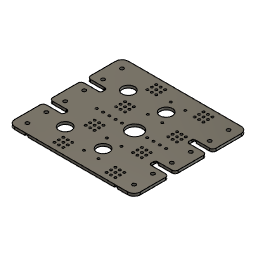
JumperTrunk_TopPlate_4mm v2 (Autodesk Fusion 360 design; units mm, degrees)
Autodesk Fusion 360 part; units mm, degrees
(part 1 of 2)
sketch "Sketch1" plane through (0, 0, 0) normal (0, 1, 0) x (1, 0, 0)
  arc A0 (10, 180) -> (0, 170) centre (10, 170) ccw
  circle A1 centre (15, 105) radius 2.75
  line L0 (171, 125) -> (194, 125)
  line L1 (199, 150) -> (199, 170)
  circle A2 centre (184, 165) radius 2.75
  arc A3 (189, 0) -> (199, 10) centre (189, 10) ccw
  line L2 (0, 150) -> (0, 170)
  circle A4 centre (184, 135) radius 2.75
  line L3 (199, 30) -> (199, 10)
  line L4 (168, 58) -> (168, 62)
  circle A5 centre (184, 105) radius 2.75
  line L5 (194, 55) -> (171, 55)
  line L6 (5, 115) -> (28, 115)
  circle A6 centre (15, 15) radius 2.75
  line L7 (0, 142) -> (0, 142.1084)
  circle A7 centre (184, 45) radius 2.75
  line L8 (0, 30) -> (0, 10)
  arc A8 (0, 10) -> (10, 0) centre (10, 10) ccw
  line L9 (31, 118) -> (31, 122)
  line L10 (5, 55) -> (28, 55)
  circle A9 centre (15, 135) radius 2.75
  line L11 (0, 82) -> (0, 82.1084)
  circle A10 centre (15, 165) radius 2.75
  line L12 (28, 65) -> (5, 65)
  line L13 (31, 58) -> (31, 62)
  circle A11 centre (15, 45) radius 2.75
  line L14 (0, 52) -> (0, 52.1084)
  line L15 (171, 65) -> (194, 65)
  line L16 (28, 125) -> (5, 125)
  circle A12 centre (184, 15) radius 2.75
  line L17 (0, 112) -> (0, 112.1084)
  line L18 (168, 118) -> (168, 122)
  line L19 (194, 115) -> (171, 115)
  line L20 (10, 0) -> (189, 0)
  line L21 (10, 180) -> (189, 180)
  arc A13 (199, 170) -> (189, 180) centre (189, 170) ccw
  circle A14 centre (70, 17) radius 1.75
  circle A15 centre (71.3, 65.26) radius 1.75
  circle A16 centre (146.23, 65.26) radius 1.75
  circle A17 centre (152.55, 17) radius 1.75
  circle A18 centre (70, 17) radius 1.75
  circle A19 centre (146.23, 65.26) radius 1.75
  circle A20 centre (71.3, 65.26) radius 1.75
  circle A21 centre (152.55, 17) radius 1.75
  circle A22 centre (71.3, 65.26) radius 1.75
  circle A23 centre (152.55, 17) radius 1.75
  circle A24 centre (146.23, 65.26) radius 1.75
  circle A25 centre (152.55, 17) radius 1.75
  circle A26 centre (70, 17) radius 1.75
  circle A27 centre (71.3, 65.26) radius 1.75
  circle A28 centre (146.23, 65.26) radius 1.75
  circle A29 centre (70, 17) radius 1.75
  circle A30 centre (64.3, 58.26) radius 1.75
  circle A31 centre (71.3, 58.26) radius 1.75
  circle A32 centre (78.3, 58.26) radius 1.75
  circle A33 centre (64.3, 65.26) radius 1.75
  circle A34 centre (78.3, 65.26) radius 1.75
  circle A35 centre (64.3, 72.26) radius 1.75
  circle A36 centre (71.3, 72.26) radius 1.75
  circle A37 centre (78.3, 72.26) radius 1.75
  circle A38 centre (63, 10) radius 1.75
  circle A39 centre (70, 10) radius 1.75
  circle A40 centre (77, 10) radius 1.75
  circle A41 centre (63, 17) radius 1.75
  circle A42 centre (77, 17) radius 1.75
  circle A43 centre (63, 24) radius 1.75
  circle A44 centre (70, 24) radius 1.75
  circle A45 centre (77, 24) radius 1.75
  circle A46 centre (139.23, 58.26) radius 1.75
  circle A47 centre (146.23, 58.26) radius 1.75
  circle A48 centre (153.23, 58.26) radius 1.75
  circle A49 centre (139.23, 65.26) radius 1.75
  circle A50 centre (153.23, 65.26) radius 1.75
  circle A51 centre (139.23, 72.26) radius 1.75
  circle A52 centre (146.23, 72.26) radius 1.75
  circle A53 centre (153.23, 72.26) radius 1.75
  circle A54 centre (145.55, 10) radius 1.75
  circle A55 centre (152.55, 10) radius 1.75
  circle A56 centre (159.55, 10) radius 1.75
  circle A57 centre (145.55, 17) radius 1.75
  circle A58 centre (159.55, 17) radius 1.75
  circle A59 centre (145.55, 24) radius 1.75
  circle A60 centre (152.55, 24) radius 1.75
  circle A61 centre (159.55, 24) radius 1.75
  circle A62 centre (159.55, 24) radius 1.75
  circle A63 centre (153.23, 65.26) radius 1.75
  circle A64 centre (71.3, 65.26) radius 1.75
  circle A65 centre (71.3, 65.26) radius 1.75
  circle A66 centre (70, 17) radius 1.75
  circle A67 centre (71.3, 72.26) radius 1.75
  circle A68 centre (146.23, 65.26) radius 1.75
  circle A69 centre (152.55, 17) radius 1.75
  circle A70 centre (63, 17) radius 1.75
  circle A71 centre (78.3, 65.26) radius 1.75
  circle A72 centre (146.23, 65.26) radius 1.75
  circle A73 centre (70, 17) radius 1.75
  circle A74 centre (159.55, 17) radius 1.75
  circle A75 centre (146.23, 72.26) radius 1.75
  circle A76 centre (153.23, 72.26) radius 1.75
  circle A77 centre (71.3, 65.26) radius 1.75
  circle A78 centre (139.23, 65.26) radius 1.75
  circle A79 centre (63, 24) radius 1.75
  circle A80 centre (77, 24) radius 1.75
  circle A81 centre (139.23, 72.26) radius 1.75
  circle A82 centre (64.3, 65.26) radius 1.75
  circle A83 centre (71.3, 65.26) radius 1.75
  circle A84 centre (71.3, 58.26) radius 1.75
  circle A85 centre (145.55, 24) radius 1.75
  circle A86 centre (152.55, 17) radius 1.75
  circle A87 centre (70, 17) radius 1.75
  circle A88 centre (70, 17) radius 1.75
  circle A89 centre (77, 17) radius 1.75
  circle A90 centre (64.3, 72.26) radius 1.75
  circle A91 centre (77, 10) radius 1.75
  circle A92 centre (152.55, 17) radius 1.75
  circle A93 centre (64.3, 58.26) radius 1.75
  circle A94 centre (145.55, 17) radius 1.75
  circle A95 centre (70, 24) radius 1.75
  circle A96 centre (63, 10) radius 1.75
  circle A97 centre (70, 10) radius 1.75
  circle A98 centre (159.55, 10) radius 1.75
  circle A99 centre (145.55, 10) radius 1.75
  circle A100 centre (152.55, 24) radius 1.75
  circle A101 centre (152.55, 10) radius 1.75
  circle A102 centre (152.55, 17) radius 1.75
  circle A103 centre (139.23, 58.26) radius 1.75
  circle A104 centre (78.3, 58.26) radius 1.75
  circle A105 centre (146.23, 65.26) radius 1.75
  circle A106 centre (146.23, 58.26) radius 1.75
  circle A107 centre (153.23, 58.26) radius 1.75
  circle A108 centre (78.3, 72.26) radius 1.75
  circle A109 centre (146.23, 65.26) radius 1.75
  circle A110 centre (145.55, 10) radius 1.75
  circle A111 centre (159.55, 10) radius 1.75
  circle A112 centre (145.55, 10) radius 1.75
  circle A113 centre (152.55, 10) radius 1.75
  circle A114 centre (78.3, 72.26) radius 1.75
  circle A115 centre (70, 17) radius 1.75
  circle A116 centre (64.3, 65.26) radius 1.75
  circle A117 centre (153.23, 65.26) radius 1.75
  circle A118 centre (71.3, 72.26) radius 1.75
  circle A119 centre (139.23, 58.26) radius 1.75
  circle A120 centre (78.3, 65.26) radius 1.75
  circle A121 centre (146.23, 65.26) radius 1.75
  circle A122 centre (78.3, 72.26) radius 1.75
  circle A123 centre (70, 17) radius 1.75
  circle A124 centre (70, 17) radius 1.75
  circle A125 centre (145.55, 17) radius 1.75
  circle A126 centre (64.3, 58.26) radius 1.75
  circle A127 centre (146.23, 65.26) radius 1.75
  circle A128 centre (152.55, 17) radius 1.75
  circle A129 centre (71.3, 65.26) radius 1.75
  circle A130 centre (70, 17) radius 1.75
  circle A131 centre (71.3, 65.26) radius 1.75
  circle A132 centre (63, 17) radius 1.75
  circle A133 centre (152.55, 17) radius 1.75
  circle A134 centre (70, 17) radius 1.75
  circle A135 centre (146.23, 72.26) radius 1.75
  circle A136 centre (146.23, 65.26) radius 1.75
  circle A137 centre (153.23, 72.26) radius 1.75
  circle A138 centre (71.3, 65.26) radius 1.75
  circle A139 centre (71.3, 72.26) radius 1.75
  circle A140 centre (64.3, 72.26) radius 1.75
  circle A141 centre (77, 24) radius 1.75
  circle A142 centre (153.23, 65.26) radius 1.75
  circle A143 centre (146.23, 72.26) radius 1.75
  circle A144 centre (70, 10) radius 1.75
  circle A145 centre (77, 10) radius 1.75
  circle A146 centre (153.23, 72.26) radius 1.75
  circle A147 centre (64.3, 65.26) radius 1.75
  circle A148 centre (159.55, 17) radius 1.75
  circle A149 centre (145.55, 24) radius 1.75
  circle A150 centre (63, 10) radius 1.75
  circle A151 centre (71.3, 58.26) radius 1.75
  circle A152 centre (70, 24) radius 1.75
  circle A153 centre (63, 24) radius 1.75
  circle A154 centre (70, 17) radius 1.75
  circle A155 centre (152.55, 17) radius 1.75
  circle A156 centre (146.23, 65.26) radius 1.75
  circle A157 centre (78.3, 58.26) radius 1.75
  circle A158 centre (146.23, 65.26) radius 1.75
  circle A159 centre (71.3, 65.26) radius 1.75
  circle A160 centre (159.55, 24) radius 1.75
  circle A161 centre (145.55, 24) radius 1.75
  circle A162 centre (153.23, 58.26) radius 1.75
  circle A163 centre (71.3, 58.26) radius 1.75
  circle A164 centre (159.55, 10) radius 1.75
  circle A165 centre (146.23, 58.26) radius 1.75
  circle A166 centre (146.23, 65.26) radius 1.75
  circle A167 centre (152.55, 17) radius 1.75
  circle A168 centre (152.55, 10) radius 1.75
  circle A169 centre (64.3, 58.26) radius 1.75
  circle A170 centre (159.55, 17) radius 1.75
  circle A171 centre (71.3, 65.26) radius 1.75
  circle A172 centre (159.55, 24) radius 1.75
  circle A173 centre (64.3, 72.26) radius 1.75
  circle A174 centre (70, 17) radius 1.75
  circle A175 centre (77, 24) radius 1.75
  circle A176 centre (71.3, 65.26) radius 1.75
  circle A177 centre (77, 10) radius 1.75
  circle A178 centre (139.23, 58.26) radius 1.75
  circle A179 centre (70, 10) radius 1.75
  circle A180 centre (152.55, 17) radius 1.75
  circle A181 centre (152.55, 24) radius 1.75
  circle A182 centre (152.55, 17) radius 1.75
  circle A183 centre (139.23, 72.26) radius 1.75
  circle A184 centre (146.23, 65.26) radius 1.75
  circle A185 centre (78.3, 65.26) radius 1.75
  circle A186 centre (139.23, 72.26) radius 1.75
  circle A187 centre (139.23, 65.26) radius 1.75
  circle A188 centre (63, 17) radius 1.75
  circle A189 centre (77, 17) radius 1.75
  circle A190 centre (146.23, 65.26) radius 1.75
  circle A191 centre (70, 17) radius 1.75
  circle A192 centre (153.23, 58.26) radius 1.75
  circle A193 centre (71.3, 65.26) radius 1.75
  circle A194 centre (152.55, 24) radius 1.75
  circle A195 centre (78.3, 58.26) radius 1.75
  circle A196 centre (77, 17) radius 1.75
  circle A197 centre (152.55, 17) radius 1.75
  circle A198 centre (139.23, 65.26) radius 1.75
  circle A199 centre (63, 24) radius 1.75
  circle A200 centre (71.3, 65.26) radius 1.75
  circle A201 centre (70, 24) radius 1.75
  circle A202 centre (152.55, 17) radius 1.75
  circle A203 centre (146.23, 58.26) radius 1.75
  circle A204 centre (63, 10) radius 1.75
  circle A205 centre (145.55, 17) radius 1.75
  circle A206 centre (64.3, 72.26) radius 1.75
  line L22 (10, 0) -> (189, 0)
  circle A207 centre (71.3, 72.26) radius 1.75
  circle A208 centre (71.3, 72.26) radius 1.75
  circle A209 centre (78.3, 72.26) radius 1.75
  circle A210 centre (64.3, 72.26) radius 1.75
  circle A211 centre (78.3, 72.26) radius 1.75
  circle A212 centre (64.3, 72.26) radius 1.75
  circle A213 centre (64.3, 72.26) radius 1.75
  circle A214 centre (139.23, 72.26) radius 1.75
  circle A215 centre (71.3, 58.26) radius 1.75
  circle A216 centre (153.23, 72.26) radius 1.75
  circle A217 centre (139.23, 72.26) radius 1.75
  circle A218 centre (152.55, 10) radius 1.75
  circle A219 centre (152.55, 17) radius 1.75
  circle A220 centre (152.55, 17) radius 1.75
  circle A221 centre (152.55, 17) radius 1.75
  circle A222 centre (71.3, 65.26) radius 1.75
  circle A223 centre (139.23, 58.26) radius 1.75
  circle A224 centre (146.23, 72.26) radius 1.75
  circle A225 centre (146.23, 72.26) radius 1.75
  circle A226 centre (71.3, 65.26) radius 1.75
  circle A227 centre (152.55, 17) radius 1.75
  circle A228 centre (145.55, 17) radius 1.75
  circle A229 centre (159.55, 10) radius 1.75
  circle A230 centre (152.55, 17) radius 1.75
  circle A231 centre (146.23, 72.26) radius 1.75
  circle A232 centre (71.3, 65.26) radius 1.75
  circle A233 centre (78.3, 58.26) radius 1.75
  circle A234 centre (71.3, 65.26) radius 1.75
  circle A235 centre (71.3, 65.26) radius 1.75
  circle A236 centre (153.23, 58.26) radius 1.75
  circle A237 centre (152.55, 10) radius 1.75
  circle A238 centre (159.55, 24) radius 1.75
  circle A239 centre (153.23, 72.26) radius 1.75
  circle A240 centre (152.55, 10) radius 1.75
  circle A241 centre (152.55, 17) radius 1.75
  circle A242 centre (159.55, 17) radius 1.75
  circle A243 centre (159.55, 17) radius 1.75
  circle A244 centre (145.55, 17) radius 1.75
  circle A245 centre (71.3, 65.26) radius 1.75
  circle A246 centre (145.55, 10) radius 1.75
  circle A247 centre (146.23, 65.26) radius 1.75
  circle A248 centre (159.55, 24) radius 1.75
  circle A249 centre (146.23, 58.26) radius 1.75
  circle A250 centre (70, 17) radius 1.75
  circle A251 centre (146.23, 65.26) radius 1.75
  circle A252 centre (159.55, 17) radius 1.75
  circle A253 centre (63, 17) radius 1.75
  circle A254 centre (70, 17) radius 1.75
  circle A255 centre (146.23, 65.26) radius 1.75
  circle A256 centre (146.23, 65.26) radius 1.75
  circle A257 centre (152.55, 17) radius 1.75
  circle A258 centre (145.55, 24) radius 1.75
  circle A259 centre (78.3, 65.26) radius 1.75
  circle A260 centre (152.55, 17) radius 1.75
  circle A261 centre (71.3, 65.26) radius 1.75
  circle A262 centre (64.3, 65.26) radius 1.75
  circle A263 centre (146.23, 65.26) radius 1.75
  circle A264 centre (146.23, 65.26) radius 1.75
  circle A265 centre (78.3, 65.26) radius 1.75
  circle A266 centre (63, 10) radius 1.75
  circle A267 centre (64.3, 58.26) radius 1.75
  circle A268 centre (70, 10) radius 1.75
  circle A269 centre (145.55, 24) radius 1.75
  circle A270 centre (152.55, 17) radius 1.75
  circle A271 centre (159.55, 24) radius 1.75
  circle A272 centre (152.55, 24) radius 1.75
  circle A273 centre (77, 17) radius 1.75
  circle A274 centre (77, 17) radius 1.75
  circle A275 centre (159.55, 17) radius 1.75
  circle A276 centre (146.23, 65.26) radius 1.75
  circle A277 centre (71.3, 65.26) radius 1.75
  circle A278 centre (153.23, 58.26) radius 1.75
  circle A279 centre (152.55, 17) radius 1.75
  circle A280 centre (139.23, 65.26) radius 1.75
  circle A281 centre (146.23, 58.26) radius 1.75
  circle A282 centre (77, 10) radius 1.75
  circle A283 centre (146.23, 65.26) radius 1.75
  circle A284 centre (77, 24) radius 1.75
  circle A285 centre (71.3, 65.26) radius 1.75
  circle A286 centre (77, 17) radius 1.75
  circle A287 centre (70, 10) radius 1.75
  circle A288 centre (64.3, 65.26) radius 1.75
  circle A289 centre (71.3, 65.26) radius 1.75
  circle A290 centre (71.3, 58.26) radius 1.75
  circle A291 centre (152.55, 17) radius 1.75
  circle A292 centre (152.55, 24) radius 1.75
  circle A293 centre (146.23, 65.26) radius 1.75
  circle A294 centre (78.3, 58.26) radius 1.75
  circle A295 centre (71.3, 65.26) radius 1.75
  circle A296 centre (78.3, 72.26) radius 1.75
  circle A297 centre (71.3, 72.26) radius 1.75
  circle A298 centre (139.23, 72.26) radius 1.75
  circle A299 centre (71.3, 72.26) radius 1.75
  circle A300 centre (78.3, 72.26) radius 1.75
  circle A301 centre (63, 24) radius 1.75
  circle A302 centre (63, 24) radius 1.75
  circle A303 centre (70, 24) radius 1.75
  circle A304 centre (70, 24) radius 1.75
  circle A305 centre (63, 17) radius 1.75
  circle A306 centre (70, 17) radius 1.75
  circle A307 centre (146.23, 65.26) radius 1.75
  circle A308 centre (77, 24) radius 1.75
  circle A309 centre (78.3, 65.26) radius 1.75
  circle A310 centre (71.3, 65.26) radius 1.75
  circle A311 centre (63, 17) radius 1.75
  circle A312 centre (64.3, 58.26) radius 1.75
  circle A313 centre (70, 17) radius 1.75
  circle A314 centre (146.23, 65.26) radius 1.75
  circle A315 centre (77, 24) radius 1.75
  circle A316 centre (64.3, 58.26) radius 1.75
  circle A317 centre (78.3, 65.26) radius 1.75
  circle A318 centre (153.23, 65.26) radius 1.75
  circle A319 centre (146.23, 65.26) radius 1.75
  circle A320 centre (146.23, 65.26) radius 1.75
  circle A321 centre (139.23, 58.26) radius 1.75
  circle A322 centre (153.23, 65.26) radius 1.75
  circle A323 centre (70, 17) radius 1.75
  circle A324 centre (64.3, 65.26) radius 1.75
  circle A325 centre (64.3, 65.26) radius 1.75
  circle A326 centre (70, 17) radius 1.75
  circle A327 centre (153.23, 58.26) radius 1.75
  circle A328 centre (70, 17) radius 1.75
  circle A329 centre (139.23, 58.26) radius 1.75
  circle A330 centre (153.23, 65.26) radius 1.75
  circle A331 centre (70, 24) radius 1.75
  circle A332 centre (139.23, 65.26) radius 1.75
  circle A333 centre (63, 17) radius 1.75
  circle A334 centre (146.23, 58.26) radius 1.75
  circle A335 centre (139.23, 65.26) radius 1.75
  circle A336 centre (146.23, 65.26) radius 1.75
  circle A337 centre (70, 17) radius 1.75
  circle A338 centre (70, 17) radius 1.75
  circle A339 centre (70, 17) radius 1.75
  circle A340 centre (70, 17) radius 1.75
  circle A341 centre (63, 24) radius 1.75
  circle A342 centre (63, 24) radius 1.75
  circle A343 centre (153.23, 65.26) radius 1.75
  circle A344 centre (77, 24) radius 1.75
  circle A345 centre (70, 17) radius 1.75
  circle A346 centre (146.23, 58.26) radius 1.75
  circle A347 centre (70, 17) radius 1.75
  circle A348 centre (70, 17) radius 1.75
  circle A349 centre (70, 24) radius 1.75
  circle A350 centre (146.23, 72.26) radius 1.75
  circle A351 centre (153.23, 72.26) radius 1.75
  circle A352 centre (153.23, 72.26) radius 1.75
  circle A353 centre (139.23, 72.26) radius 1.75
  circle A354 centre (153.23, 58.26) radius 1.75
  circle A355 centre (139.23, 58.26) radius 1.75
  circle A356 centre (145.55, 17) radius 1.75
  circle A357 centre (71.3, 65.26) radius 1.75
  circle A358 centre (77, 10) radius 1.75
  circle A359 centre (146.23, 65.26) radius 1.75
  circle A360 centre (145.55, 24) radius 1.75
  circle A361 centre (145.55, 10) radius 1.75
  circle A362 centre (71.3, 58.26) radius 1.75
  circle A363 centre (77, 17) radius 1.75
  circle A364 centre (70, 17) radius 1.75
  circle A365 centre (78.3, 58.26) radius 1.75
  circle A366 centre (70, 10) radius 1.75
  circle A367 centre (139.23, 65.26) radius 1.75
  circle A368 centre (152.55, 24) radius 1.75
  circle A369 centre (152.55, 17) radius 1.75
  circle A370 centre (159.55, 10) radius 1.75
  circle A371 centre (152.55, 17) radius 1.75
  circle A372 centre (77, 10) radius 1.75
  circle A373 centre (70, 10) radius 1.75
  circle A374 centre (78.3, 58.26) radius 1.75
  circle A375 centre (145.55, 24) radius 1.75
  circle A376 centre (71.3, 65.26) radius 1.75
  circle A377 centre (145.55, 10) radius 1.75
  circle A378 centre (152.55, 24) radius 1.75
  circle A379 centre (77, 10) radius 1.75
  circle A380 centre (70, 17) radius 1.75
  circle A381 centre (71.3, 65.26) radius 1.75
  circle A382 centre (63, 10) radius 1.75
  circle A383 centre (146.23, 65.26) radius 1.75
  circle A384 centre (63, 10) radius 1.75
  circle A385 centre (71.3, 65.26) radius 1.75
  circle A386 centre (152.55, 17) radius 1.75
  circle A387 centre (152.55, 17) radius 1.75
  circle A388 centre (152.55, 10) radius 1.75
  circle A389 centre (64.3, 58.26) radius 1.75
  circle A390 centre (63, 10) radius 1.75
  circle A391 centre (145.55, 17) radius 1.75
  circle A392 centre (159.55, 10) radius 1.75
  circle A393 centre (159.55, 24) radius 1.75
  circle A394 centre (152.55, 17) radius 1.75
  circle A395 centre (71.3, 58.26) radius 1.75
  circle A396 centre (145.55, 10) radius 1.75
  circle A397 centre (159.55, 10) radius 1.75
  circle A398 centre (64.3, 156) radius 1.75
  circle A399 centre (139.23, 170) radius 1.75
  circle A400 centre (145.55, 121.74) radius 1.75
  circle A401 centre (64.3, 170) radius 1.75
  circle A402 centre (145.55, 121.74) radius 1.75
  circle A403 centre (64.3, 170) radius 1.75
  circle A404 centre (145.55, 121.74) radius 1.75
  circle A405 centre (64.3, 170) radius 1.75
  circle A406 centre (145.55, 121.74) radius 1.75
  circle A407 centre (139.23, 163) radius 1.75
  circle A408 centre (139.23, 163) radius 1.75
  circle A409 centre (139.23, 170) radius 1.75
  circle A410 centre (152.55, 121.74) radius 1.75
  circle A411 centre (64.3, 170) radius 1.75
  circle A412 centre (64.3, 170) radius 1.75
  circle A413 centre (64.3, 163) radius 1.75
  circle A414 centre (152.55, 121.74) radius 1.75
  circle A415 centre (139.23, 156) radius 1.75
  circle A416 centre (64.3, 156) radius 1.75
  circle A417 centre (152.55, 121.74) radius 1.75
  circle A418 centre (145.55, 121.74) radius 1.75
  circle A419 centre (64.3, 156) radius 1.75
  circle A420 centre (145.55, 121.74) radius 1.75
  circle A421 centre (64.3, 156) radius 1.75
  circle A422 centre (139.23, 163) radius 1.75
  circle A423 centre (64.3, 170) radius 1.75
  circle A424 centre (64.3, 163) radius 1.75
  circle A425 centre (139.23, 156) radius 1.75
  circle A426 centre (145.55, 121.74) radius 1.75
  circle A427 centre (159.55, 107.74) radius 1.75
  circle A428 centre (153.23, 170) radius 1.75
  circle A429 centre (152.55, 107.74) radius 1.75
  circle A430 centre (152.55, 114.74) radius 1.75
  circle A431 centre (153.23, 170) radius 1.75
  circle A432 centre (71.3, 163) radius 1.75
  circle A433 centre (77, 121.74) radius 1.75
  circle A434 centre (152.55, 114.74) radius 1.75
  circle A435 centre (159.55, 107.74) radius 1.75
  circle A436 centre (153.23, 156) radius 1.75
  circle A437 centre (159.55, 107.74) radius 1.75
  circle A438 centre (159.55, 107.74) radius 1.75
  circle A439 centre (159.55, 114.74) radius 1.75
  circle A440 centre (77, 121.74) radius 1.75
  circle A441 centre (159.55, 114.74) radius 1.75
  circle A442 centre (152.55, 114.74) radius 1.75
  circle A443 centre (152.55, 107.74) radius 1.75
  circle A444 centre (71.3, 163) radius 1.75
  circle A445 centre (152.55, 107.74) radius 1.75
  circle A446 centre (71.3, 163) radius 1.75
  circle A447 centre (152.55, 114.74) radius 1.75
  circle A448 centre (77, 121.74) radius 1.75
  circle A449 centre (152.55, 114.74) radius 1.75
  circle A450 centre (153.23, 163) radius 1.75
  circle A451 centre (152.55, 114.74) radius 1.75
  circle A452 centre (152.55, 107.74) radius 1.75
  circle A453 centre (145.55, 114.74) radius 1.75
  circle A454 centre (145.55, 114.74) radius 1.75
  circle A455 centre (146.23, 156) radius 1.75
  circle A456 centre (71.3, 156) radius 1.75
  circle A457 centre (71.3, 156) radius 1.75
  circle A458 centre (146.23, 156) radius 1.75
  circle A459 centre (145.55, 107.74) radius 1.75
  circle A460 centre (70, 121.74) radius 1.75
  circle A461 centre (63, 121.74) radius 1.75
  circle A462 centre (145.55, 114.74) radius 1.75
  circle A463 centre (145.55, 107.74) radius 1.75
  circle A464 centre (146.23, 156) radius 1.75
  circle A465 centre (145.55, 114.74) radius 1.75
  circle A466 centre (145.55, 107.74) radius 1.75
  circle A467 centre (146.23, 156) radius 1.75
  circle A468 centre (63, 121.74) radius 1.75
  circle A469 centre (71.3, 156) radius 1.75
  circle A470 centre (146.23, 156) radius 1.75
  circle A471 centre (71.3, 163) radius 1.75
  circle A472 centre (152.55, 114.74) radius 1.75
  circle A473 centre (146.23, 163) radius 1.75
  circle A474 centre (78.3, 156) radius 1.75
  circle A475 centre (153.23, 163) radius 1.75
  circle A476 centre (146.23, 163) radius 1.75
  circle A477 centre (146.23, 163) radius 1.75
  circle A478 centre (63, 107.74) radius 1.75
  circle A479 centre (78.3, 163) radius 1.75
  circle A480 centre (71.3, 163) radius 1.75
  circle A481 centre (78.3, 163) radius 1.75
  circle A482 centre (63, 114.74) radius 1.75
  circle A483 centre (78.3, 163) radius 1.75
  circle A484 centre (71.3, 163) radius 1.75
  circle A485 centre (146.23, 163) radius 1.75
  circle A486 centre (63, 107.74) radius 1.75
  circle A487 centre (78.3, 156) radius 1.75
  circle A488 centre (78.3, 170) radius 1.75
  circle A489 centre (71.3, 163) radius 1.75
  circle A490 centre (71.3, 163) radius 1.75
  circle A491 centre (63, 114.74) radius 1.75
  circle A492 centre (71.3, 170) radius 1.75
  circle A493 centre (71.3, 163) radius 1.75
  circle A494 centre (70, 114.74) radius 1.75
  circle A495 centre (71.3, 163) radius 1.75
  circle A496 centre (146.23, 163) radius 1.75
  circle A497 centre (146.23, 163) radius 1.75
  circle A498 centre (153.23, 163) radius 1.75
  circle A499 centre (78.3, 170) radius 1.75
  circle A500 centre (63, 114.74) radius 1.75
  circle A501 centre (146.23, 163) radius 1.75
  circle A502 centre (78.3, 156) radius 1.75
  circle A503 centre (146.23, 163) radius 1.75
  circle A504 centre (146.23, 163) radius 1.75
  circle A505 centre (78.3, 163) radius 1.75
  circle A506 centre (63, 107.74) radius 1.75
  circle A507 centre (71.3, 170) radius 1.75
  circle A508 centre (152.55, 114.74) radius 1.75
  circle A509 centre (71.3, 170) radius 1.75
  circle A510 centre (71.3, 170) radius 1.75
  circle A511 centre (71.3, 163) radius 1.75
  circle A512 centre (71.3, 163) radius 1.75
  circle A513 centre (153.23, 156) radius 1.75
  circle A514 centre (71.3, 170) radius 1.75
  circle A515 centre (71.3, 163) radius 1.75
  circle A516 centre (63, 107.74) radius 1.75
  circle A517 centre (153.23, 170) radius 1.75
  circle A518 centre (146.23, 163) radius 1.75
  circle A519 centre (153.23, 170) radius 1.75
  circle A520 centre (71.3, 163) radius 1.75
  circle A521 centre (152.55, 114.74) radius 1.75
  circle A522 centre (153.23, 163) radius 1.75
  circle A523 centre (146.23, 163) radius 1.75
  circle A524 centre (71.3, 170) radius 1.75
  circle A525 centre (152.55, 114.74) radius 1.75
  circle A526 centre (63, 114.74) radius 1.75
  circle A527 centre (146.23, 163) radius 1.75
  circle A528 centre (63, 114.74) radius 1.75
  circle A529 centre (146.23, 163) radius 1.75
  circle A530 centre (71.3, 163) radius 1.75
  circle A531 centre (152.55, 114.74) radius 1.75
  circle A532 centre (146.23, 163) radius 1.75
  circle A533 centre (71.3, 163) radius 1.75
  circle A534 centre (153.23, 156) radius 1.75
  circle A535 centre (153.23, 156) radius 1.75
  circle A536 centre (63, 107.74) radius 1.75
  circle A537 centre (153.23, 156) radius 1.75
  circle A538 centre (146.23, 163) radius 1.75
  circle A539 centre (71.3, 170) radius 1.75
  circle A540 centre (152.55, 114.74) radius 1.75
  circle A541 centre (152.55, 114.74) radius 1.75
  circle A542 centre (152.55, 107.74) radius 1.75
  circle A543 centre (146.23, 156) radius 1.75
  circle A544 centre (70, 121.74) radius 1.75
  circle A545 centre (152.55, 114.74) radius 1.75
  circle A546 centre (70, 121.74) radius 1.75
  circle A547 centre (159.55, 114.74) radius 1.75
  circle A548 centre (152.55, 114.74) radius 1.75
  circle A549 centre (146.23, 156) radius 1.75
  circle A550 centre (152.55, 114.74) radius 1.75
  circle A551 centre (159.55, 107.74) radius 1.75
  circle A552 centre (70, 121.74) radius 1.75
  circle A553 centre (159.55, 114.74) radius 1.75
  circle A554 centre (159.55, 114.74) radius 1.75
  circle A555 centre (159.55, 114.74) radius 1.75
  circle A556 centre (159.55, 114.74) radius 1.75
  circle A557 centre (70, 121.74) radius 1.75
  circle A558 centre (70, 121.74) radius 1.75
  circle A559 centre (145.55, 107.74) radius 1.75
  circle A560 centre (159.55, 114.74) radius 1.75
  circle A561 centre (152.55, 107.74) radius 1.75
  circle A562 centre (70, 121.74) radius 1.75
  circle A563 centre (152.55, 114.74) radius 1.75
  circle A564 centre (70, 121.74) radius 1.75
  circle A565 centre (146.23, 156) radius 1.75
  circle A566 centre (152.55, 114.74) radius 1.75
  circle A567 centre (64.3, 163) radius 1.75
  circle A568 centre (139.23, 156) radius 1.75
  circle A569 centre (64.3, 156) radius 1.75
  circle A570 centre (139.23, 163) radius 1.75
  circle A571 centre (64.3, 170) radius 1.75
  circle A572 centre (145.55, 121.74) radius 1.75
  circle A573 centre (139.23, 163) radius 1.75
  circle A574 centre (64.3, 156) radius 1.75
  circle A575 centre (139.23, 170) radius 1.75
  circle A576 centre (64.3, 163) radius 1.75
  circle A577 centre (78.3, 163) radius 1.75
  circle A578 centre (78.3, 156) radius 1.75
  circle A579 centre (71.3, 163) radius 1.75
  circle A580 centre (78.3, 163) radius 1.75
  circle A581 centre (63, 107.74) radius 1.75
  circle A582 centre (146.23, 163) radius 1.75
  circle A583 centre (63, 114.74) radius 1.75
  circle A584 centre (78.3, 170) radius 1.75
  circle A585 centre (78.3, 170) radius 1.75
  circle A586 centre (146.23, 163) radius 1.75
  circle A587 centre (63, 107.74) radius 1.75
  circle A588 centre (146.23, 163) radius 1.75
  circle A589 centre (78.3, 156) radius 1.75
  circle A590 centre (78.3, 170) radius 1.75
  circle A591 centre (78.3, 170) radius 1.75
  circle A592 centre (63, 114.74) radius 1.75
  circle A593 centre (77, 114.74) radius 1.75
  circle A594 centre (146.23, 163) radius 1.75
  circle A595 centre (78.3, 170) radius 1.75
  circle A596 centre (78.3, 170) radius 1.75
  circle A597 centre (71.3, 163) radius 1.75
  circle A598 centre (71.3, 163) radius 1.75
  circle A599 centre (146.23, 163) radius 1.75
  circle A600 centre (63, 114.74) radius 1.75
  circle A601 centre (63, 107.74) radius 1.75
  circle A602 centre (70, 114.74) radius 1.75
  circle A603 centre (70, 114.74) radius 1.75
  circle A604 centre (70, 114.74) radius 1.75
  circle A605 centre (70, 114.74) radius 1.75
  circle A606 centre (70, 114.74) radius 1.75
  circle A607 centre (70, 114.74) radius 1.75
  circle A608 centre (77, 114.74) radius 1.75
  circle A609 centre (70, 114.74) radius 1.75
  circle A610 centre (70, 114.74) radius 1.75
  circle A611 centre (77, 114.74) radius 1.75
  circle A612 centre (70, 114.74) radius 1.75
  circle A613 centre (70, 114.74) radius 1.75
  circle A614 centre (70, 107.74) radius 1.75
  circle A615 centre (70, 107.74) radius 1.75
  circle A616 centre (77, 114.74) radius 1.75
  circle A617 centre (70, 114.74) radius 1.75
  circle A618 centre (70, 114.74) radius 1.75
  circle A619 centre (78.3, 156) radius 1.75
  circle A620 centre (77, 114.74) radius 1.75
  circle A621 centre (70, 114.74) radius 1.75
  circle A622 centre (70, 114.74) radius 1.75
  circle A623 centre (70, 114.74) radius 1.75
  circle A624 centre (70, 114.74) radius 1.75
  circle A625 centre (77, 107.74) radius 1.75
  circle A626 centre (70, 114.74) radius 1.75
  circle A627 centre (78.3, 163) radius 1.75
  circle A628 centre (77, 114.74) radius 1.75
  circle A629 centre (70, 114.74) radius 1.75
  circle A630 centre (70, 114.74) radius 1.75
  circle A631 centre (78.3, 156) radius 1.75
  circle A632 centre (70, 107.74) radius 1.75
  circle A633 centre (70, 114.74) radius 1.75
  circle A634 centre (70, 114.74) radius 1.75
  circle A635 centre (78.3, 163) radius 1.75
  circle A636 centre (70, 114.74) radius 1.75
  circle A637 centre (70, 114.74) radius 1.75
  circle A638 centre (70, 114.74) radius 1.75
  circle A639 centre (78.3, 156) radius 1.75
  circle A640 centre (64.3, 163) radius 1.75
  circle A641 centre (139.23, 163) radius 1.75
  circle A642 centre (159.55, 121.74) radius 1.75
  circle A643 centre (145.55, 107.74) radius 1.75
  circle A644 centre (139.23, 170) radius 1.75
  circle A645 centre (64.3, 156) radius 1.75
  circle A646 centre (139.23, 163) radius 1.75
  circle A647 centre (159.55, 121.74) radius 1.75
  circle A648 centre (145.55, 107.74) radius 1.75
  circle A649 centre (139.23, 156) radius 1.75
  circle A650 centre (159.55, 121.74) radius 1.75
  circle A651 centre (145.55, 114.74) radius 1.75
  circle A652 centre (63, 121.74) radius 1.75
  circle A653 centre (139.23, 156) radius 1.75
  circle A654 centre (159.55, 121.74) radius 1.75
  circle A655 centre (159.55, 121.74) radius 1.75
  circle A656 centre (71.3, 156) radius 1.75
  circle A657 centre (71.3, 156) radius 1.75
  circle A658 centre (139.23, 170) radius 1.75
  circle A659 centre (145.55, 114.74) radius 1.75
  circle A660 centre (145.55, 107.74) radius 1.75
  circle A661 centre (139.23, 170) radius 1.75
  circle A662 centre (63, 121.74) radius 1.75
  circle A663 centre (71.3, 156) radius 1.75
  circle A664 centre (145.55, 114.74) radius 1.75
  circle A665 centre (159.55, 121.74) radius 1.75
  circle A666 centre (63, 121.74) radius 1.75
  circle A667 centre (159.55, 121.74) radius 1.75
  circle A668 centre (71.3, 156) radius 1.75
  circle A669 centre (71.3, 156) radius 1.75
  circle A670 centre (145.55, 107.74) radius 1.75
  circle A671 centre (139.23, 170) radius 1.75
  circle A672 centre (63, 121.74) radius 1.75
  circle A673 centre (145.55, 114.74) radius 1.75
  circle A674 centre (63, 121.74) radius 1.75
  circle A675 centre (63, 121.74) radius 1.75
  circle A676 centre (159.55, 121.74) radius 1.75
  circle A677 centre (77, 121.74) radius 1.75
  circle A678 centre (152.55, 114.74) radius 1.75
  circle A679 centre (153.23, 156) radius 1.75
  circle A680 centre (146.23, 170) radius 1.75
  circle A681 centre (152.55, 114.74) radius 1.75
  circle A682 centre (71.3, 163) radius 1.75
  circle A683 centre (71.3, 163) radius 1.75
  circle A684 centre (146.23, 163) radius 1.75
  circle A685 centre (71.3, 163) radius 1.75
  circle A686 centre (153.23, 156) radius 1.75
  circle A687 centre (71.3, 170) radius 1.75
  circle A688 centre (146.23, 163) radius 1.75
  circle A689 centre (153.23, 163) radius 1.75
  circle A690 centre (153.23, 170) radius 1.75
  circle A691 centre (152.55, 114.74) radius 1.75
  circle A692 centre (153.23, 170) radius 1.75
  circle A693 centre (71.3, 163) radius 1.75
  circle A694 centre (159.55, 107.74) radius 1.75
  circle A695 centre (146.23, 170) radius 1.75
  circle A696 centre (152.55, 114.74) radius 1.75
  circle A697 centre (71.3, 163) radius 1.75
  circle A698 centre (153.23, 163) radius 1.75
  circle A699 centre (146.23, 163) radius 1.75
  circle A700 centre (146.23, 163) radius 1.75
  circle A701 centre (152.55, 114.74) radius 1.75
  circle A702 centre (70, 114.74) radius 1.75
  circle A703 centre (152.55, 114.74) radius 1.75
  circle A704 centre (146.23, 163) radius 1.75
  circle A705 centre (146.23, 163) radius 1.75
  circle A706 centre (153.23, 170) radius 1.75
  circle A707 centre (71.3, 163) radius 1.75
  circle A708 centre (152.55, 114.74) radius 1.75
  circle A709 centre (153.23, 163) radius 1.75
  circle A710 centre (146.23, 163) radius 1.75
  circle A711 centre (71.3, 163) radius 1.75
  circle A712 centre (152.55, 114.74) radius 1.75
  circle A713 centre (146.23, 163) radius 1.75
  circle A714 centre (146.23, 163) radius 1.75
  circle A715 centre (152.55, 114.74) radius 1.75
  circle A716 centre (71.3, 163) radius 1.75
  circle A717 centre (146.23, 170) radius 1.75
  circle A718 centre (152.55, 107.74) radius 1.75
  circle A719 centre (71.3, 163) radius 1.75
  circle A720 centre (152.55, 114.74) radius 1.75
  circle A721 centre (159.55, 107.74) radius 1.75
  circle A722 centre (77, 121.74) radius 1.75
  circle A723 centre (152.55, 114.74) radius 1.75
  circle A724 centre (152.55, 114.74) radius 1.75
  circle A725 centre (146.23, 170) radius 1.75
  circle A726 centre (153.23, 163) radius 1.75
  circle A727 centre (146.23, 163) radius 1.75
  circle A728 centre (159.55, 107.74) radius 1.75
  circle A729 centre (71.3, 163) radius 1.75
  circle A730 centre (146.23, 163) radius 1.75
  circle A731 centre (153.23, 170) radius 1.75
  circle A732 centre (71.3, 163) radius 1.75
  circle A733 centre (71.3, 163) radius 1.75
  circle A734 centre (77, 121.74) radius 1.75
  circle A735 centre (152.55, 114.74) radius 1.75
  circle A736 centre (146.23, 170) radius 1.75
  circle A737 centre (71.3, 163) radius 1.75
  circle A738 centre (153.23, 156) radius 1.75
  circle A739 centre (146.23, 170) radius 1.75
  circle A740 centre (146.23, 170) radius 1.75
  circle A741 centre (146.23, 170) radius 1.75
  circle A742 centre (77, 121.74) radius 1.75
  circle A743 centre (152.55, 114.74) radius 1.75
  circle A744 centre (152.55, 107.74) radius 1.75
  circle A745 centre (146.23, 163) radius 1.75
  circle A746 centre (77, 121.74) radius 1.75
  circle A747 centre (64.3, 156) radius 1.75
  circle A748 centre (139.23, 163) radius 1.75
  circle A749 centre (139.23, 156) radius 1.75
  circle A750 centre (152.55, 121.74) radius 1.75
  circle A751 centre (64.3, 163) radius 1.75
  circle A752 centre (64.3, 163) radius 1.75
  circle A753 centre (139.23, 156) radius 1.75
  circle A754 centre (77, 107.74) radius 1.75
  circle A755 centre (70, 107.74) radius 1.75
  circle A756 centre (70, 107.74) radius 1.75
  circle A757 centre (77, 114.74) radius 1.75
  circle A758 centre (70, 114.74) radius 1.75
  circle A759 centre (70, 114.74) radius 1.75
  circle A760 centre (77, 107.74) radius 1.75
  circle A761 centre (70, 114.74) radius 1.75
  circle A762 centre (70, 107.74) radius 1.75
  circle A763 centre (70, 107.74) radius 1.75
  circle A764 centre (77, 107.74) radius 1.75
  circle A765 centre (77, 107.74) radius 1.75
  circle A766 centre (70, 107.74) radius 1.75
  circle A767 centre (70, 114.74) radius 1.75
  circle A768 centre (77, 107.74) radius 1.75
  circle A769 centre (70, 114.74) radius 1.75
  circle A770 centre (77, 107.74) radius 1.75
  circle A771 centre (70, 114.74) radius 1.75
  circle A772 centre (77, 114.74) radius 1.75
  circle A773 centre (77, 107.74) radius 1.75
  circle A774 centre (152.55, 121.74) radius 1.75
  circle A775 centre (139.23, 170) radius 1.75
  circle A776 centre (64.3, 170) radius 1.75
  circle A777 centre (152.55, 121.74) radius 1.75
  circle A778 centre (139.23, 156) radius 1.75
  circle A779 centre (152.55, 121.74) radius 1.75
  circle A780 centre (64.3, 163) radius 1.75
  circle A781 centre (152.55, 121.74) radius 1.75
  arc A782 (31, 122) -> (28, 125) centre (28, 122) ccw
  arc A783 (28, 115) -> (31, 118) centre (28, 118) ccw
  arc A784 (31, 62) -> (28, 65) centre (28, 62) ccw
  arc A785 (28, 55) -> (31, 58) centre (28, 58) ccw
  arc A786 (171, 125) -> (168, 122) centre (171, 122) ccw
  arc A787 (168, 118) -> (171, 115) centre (171, 118) ccw
  arc A788 (171, 65) -> (168, 62) centre (171, 62) ccw
  arc A789 (168, 58) -> (171, 55) centre (171, 58) ccw
  circle A790 centre (15, 75) radius 2.75
  line L23 (0, 150) -> (0, 130)
  line L24 (0, 110) -> (0, 70)
  line L25 (0, 50) -> (0, 30)
  arc A791 (5, 55) -> (0, 50) centre (5, 50) ccw
  arc A792 (0, 70) -> (5, 65) centre (5, 70) ccw
  arc A793 (5, 115) -> (0, 110) centre (5, 110) ccw
  arc A794 (0, 130) -> (5, 125) centre (5, 130) ccw
  circle A795 centre (184, 75) radius 2.75
  line L26 (199, 30) -> (199, 50)
  line L27 (199, 70) -> (199, 110)
  line L28 (199, 130) -> (199, 150)
  arc A796 (194, 125) -> (199, 130) centre (194, 130) ccw
  arc A797 (199, 110) -> (194, 115) centre (194, 110) ccw
  arc A798 (194, 65) -> (199, 70) centre (194, 70) ccw
  arc A799 (199, 50) -> (194, 55) centre (194, 50) ccw
  point P0 (169, 130)
  point P1 (0, 110.1084)
  dimension "d1" = 5.5
  dimension "d4" = 10
  dimension "d5" = 10
  dimension "d6" = 10
  dimension "d7" = 10
  dimension "d116" = 82.55
  dimension "d121" = 7
  dimension "d122" = 7
  dimension "d125" = 7
  dimension "d126" = 7
  dimension "d129" = 7
  dimension "d130" = 7
  dimension "d133" = 7
  dimension "d134" = 7
  dimension "d137" = 7
  dimension "d138" = 7
  dimension "d141" = 7
  dimension "d142" = 7
  dimension "d145" = 7
  dimension "d146" = 7
  dimension "d149" = 7
  dimension "d150" = 7
  dimension "d152" = 82.55
  dimension "d196" = 7
  dimension "d197" = 7
  dimension "d200" = 7
  dimension "d201" = 7
  dimension "d204" = 7
  dimension "d205" = 7
  dimension "d208" = 7
  dimension "d209" = 7
  dimension "d212" = 7
  dimension "d213" = 7
  dimension "d216" = 7
  dimension "d217" = 7
  dimension "d220" = 7
  dimension "d221" = 7
  dimension "d224" = 7
  dimension "d225" = 7
  dimension "d227" = 82.55
  dimension "d230" = 82.55
  dimension "d232" = 180
  dimension "d238" = 7
  dimension "d239" = 7
  dimension "d242" = 7
  dimension "d243" = 7
  dimension "d246" = 7
  dimension "d247" = 7
  dimension "d250" = 7
  dimension "d251" = 7
  dimension "d254" = 7
  dimension "d255" = 7
  dimension "d258" = 7
  dimension "d259" = 7
  dimension "d262" = 7
  dimension "d263" = 7
  dimension "d266" = 7
  dimension "d267" = 7
  dimension "d270" = 7
  dimension "d271" = 7
  dimension "d274" = 7
  dimension "d275" = 7
  dimension "d278" = 7
  dimension "d279" = 7
  dimension "d282" = 7
  dimension "d283" = 7
  dimension "d286" = 7
  dimension "d287" = 7
  dimension "d290" = 7
  dimension "d291" = 7
  dimension "d294" = 7
  dimension "d295" = 7
  dimension "d298" = 7
  dimension "d299" = 7
  dimension "d303" = 82.55
  dimension "d305" = 74.93
  dimension "d306" = 82.55
  dimension "d310" = 82.55
  dimension "d313" = 82.55
  dimension "d319" = 48.26
  dimension "d322" = 7
  dimension "d323" = 7
  dimension "d326" = 7
  dimension "d327" = 7
  dimension "d330" = 7
  dimension "d331" = 7
  dimension "d334" = 7
  dimension "d335" = 7
  dimension "d338" = 7
  dimension "d339" = 7
  dimension "d342" = 7
  dimension "d343" = 7
  dimension "d346" = 7
  dimension "d347" = 7
  dimension "d350" = 7
  dimension "d351" = 7
  dimension "d354" = 7
  dimension "d355" = 7
  dimension "d358" = 7
  dimension "d359" = 7
  dimension "d362" = 7
  dimension "d363" = 7
  dimension "d366" = 7
  dimension "d367" = 7
  dimension "d370" = 7
  dimension "d371" = 7
  dimension "d374" = 7
  dimension "d375" = 7
  dimension "d378" = 7
  dimension "d379" = 7
  dimension "d382" = 7
  dimension "d383" = 7
  dimension "d386" = 7
  dimension "d387" = 7
  dimension "d390" = 7
  dimension "d391" = 7
  dimension "d394" = 7
  dimension "d395" = 7
  dimension "d398" = 7
  dimension "d399" = 7
  dimension "d402" = 7
  dimension "d403" = 7
  dimension "d406" = 7
  dimension "d407" = 7
  dimension "d410" = 7
  dimension "d411" = 7
  dimension "d414" = 7
  dimension "d415" = 7
  dimension "d418" = 7
  dimension "d419" = 7
  dimension "d422" = 7
  dimension "d423" = 7
  dimension "d426" = 7
  dimension "d427" = 7
  dimension "d430" = 7
  dimension "d431" = 7
  dimension "d434" = 7
  dimension "d435" = 7
  dimension "d438" = 7
  dimension "d439" = 7
  dimension "d442" = 7
  dimension "d443" = 7
  dimension "d446" = 7
  dimension "d447" = 7
  dimension "d448" = 82.55
  dimension "d449" = 82.55
  dimension "d450" = 82.55
  dimension "d451" = 82.55
  dimension "d452" = 82.55
  dimension "d453" = 74.93
  dimension "d454" = 82.55
  dimension "d455" = 82.55
  dimension "d456" = 82.55
  dimension "d457" = 48.26
  dimension "d459" = 10
  dimension "d460" = 10
  dimension "d461" = 35.48
  dimension "d538" = 3
  dimension "d539" = 3
  dimension "d540" = 3
  dimension "d541" = 3
  dimension "d542" = 3
  dimension "d543" = 3
  dimension "d544" = 3
  dimension "d545" = 3
  dimension "d571" = 15
  dimension "d572" = 30
  dimension "d573" = 15
  dimension "d574" = 30
  dimension "d575" = 30
  dimension "d576" = 5.5
  dimension "d578" = 30
  dimension "d579" = 5
  dimension "d580" = 5
  dimension "d581" = 5
  dimension "d582" = 5
  dimension "d583" = 15
  dimension "d584" = 30
  dimension "d585" = 30
  dimension "d586" = 15
  dimension "d587" = 30
  dimension "d588" = 5.5
  dimension "d591" = 30
  dimension "d592" = 5
  dimension "d593" = 5
  dimension "d594" = 5
  dimension "d595" = 5
  constraint perpendicular L3 L20
  constraint tangent A0 L2
  constraint tangent A0 L21
  constraint tangent L1 A13
  constraint tangent L21 A13
  constraint tangent A3 L3
  constraint tangent A3 L20
  constraint tangent L8 A8
  constraint tangent A8 L20
  constraint tangent L16 A782
  constraint tangent L9 A782
  constraint tangent L6 A783
  constraint tangent L9 A783
  constraint tangent L12 A784
  constraint tangent L13 A784
  constraint tangent L10 A785
  constraint tangent L13 A785
  constraint tangent L0 A786
  constraint tangent L18 A786
  constraint tangent L18 A787
  constraint tangent L19 A787
  constraint tangent L4 A788
  constraint tangent L15 A788
  constraint tangent L5 A789
  constraint tangent L4 A789
  constraint parallel L7 L23
  constraint perpendicular L6 L24
  constraint perpendicular L10 L25
  constraint tangent L25 A791
  constraint coincident L10.start A791.start
  constraint tangent L24 A792
  constraint coincident L12.end A792.end
  constraint tangent L24 A793
  constraint coincident L6.start A793.start
  constraint tangent L23 A794
  constraint coincident L16.end A794.end
  constraint parallel L3 L26
  constraint perpendicular L0 L28
  constraint tangent L28 A796
  constraint coincident L0.end A796.start
  constraint tangent L27 A797
  constraint coincident L19.start A797.end
  constraint tangent L27 A798
  constraint coincident L15.end A798.start
  constraint tangent L26 A799
  constraint coincident L5.start A799.end
  measures "d1" diameter of A12
  measures "d4" radius of A0
  measures "d5" radius of A13
  measures "d6" radius of A3
  measures "d7" radius of A8
  measures "d116" distance of A17.centre A14.centre
  measures "d152" distance of A14.centre A17.centre
  measures "d227" distance of A14.centre A17.centre
  measures "d230" distance of A14.centre A17.centre
  measures "d232" distance of L20 L21
  measures "d303" distance of A14.centre A17.centre
  measures "d305" distance of A16.centre A15.centre
  measures "d306" distance of A14.centre A17.centre
  measures "d310" distance of A14.centre A17.centre
  measures "d313" distance of A14.centre A17.centre
  measures "d319" vertical distance of A14.centre A15.centre
  measures "d448" distance of A494.centre A430.centre
  measures "d449" distance of A494.centre A430.centre
  measures "d450" distance of A494.centre A430.centre
  measures "d451" distance of A494.centre A430.centre
  measures "d452" distance of A494.centre A430.centre
  measures "d453" distance of A432.centre A473.centre
  measures "d454" distance of A430.centre A494.centre
  measures "d455" distance of A430.centre A494.centre
  measures "d456" distance of A494.centre A430.centre
  measures "d457" vertical distance of A494.centre A432.centre
  measures "d459" distance of L20 A56.centre
  measures "d460" distance of L21 A428.centre
  measures "d461" vertical distance of A53.centre A427.centre
  measures "d538" radius of A782
  measures "d539" radius of A783
  measures "d540" radius of A784
  measures "d541" radius of A785
  measures "d542" radius of A786
  measures "d543" radius of A787
  measures "d544" radius of A788
  measures "d545" radius of A789
  measures "d571" distance of A10.centre L21
  measures "d572" distance of A9.centre A10.centre
  measures "d573" distance of A6.centre L20
  measures "d574" distance of A11.centre A6.centre A430.centre
  measures "d575" distance of A9.centre A1.centre A430.centre
  measures "d576" diameter of A790
  measures "d578" distance of A11.centre A790.centre
  measures "d579" radius of A791
  measures "d580" radius of A792
  measures "d581" radius of A793
  measures "d582" radius of A794
  measures "d583" distance of A2.centre L21
  measures "d584" distance of A2.centre A4.centre
  measures "d585" distance of A5.centre A4.centre
  measures "d586" distance of A12.centre L22
  measures "d587" distance of A12.centre A7.centre
  measures "d588" diameter of A795
  measures "d591" distance of A5.centre A795.centre
  measures "d592" radius of A796
  measures "d593" radius of A797
  measures "d594" radius of A798
  measures "d595" radius of A799